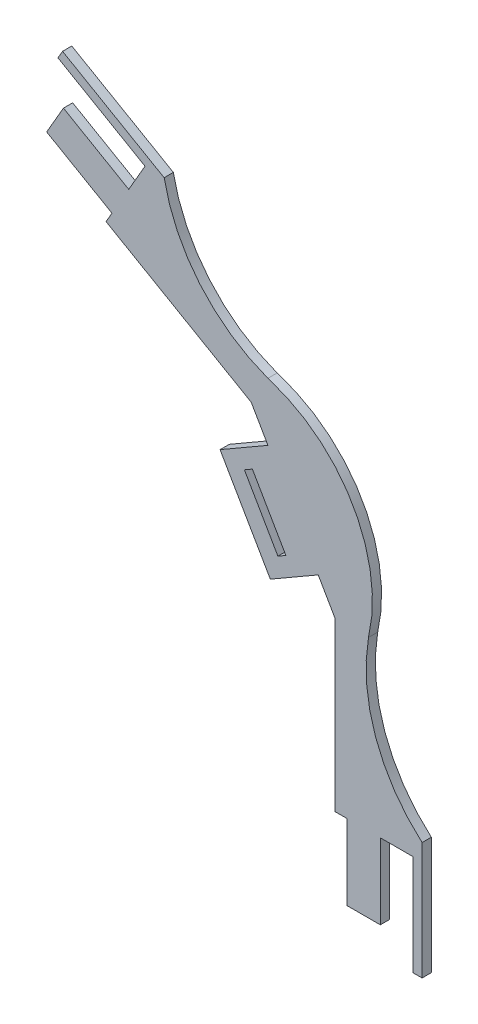
# Autodesk Inventor part: brazos
Saved by Autodesk Inventor 2015 (Build 190159000, 159)
## iProperties
Created: 2017-10-02
Part Number: brazos
Material: Generic
Document SubType Name: Modeling
Designer: macbook
Density: 1 g/cm^3
Appearance: Default
Author: macbook
Autodesk Inventor part; units mm, degrees
ref_plane "YZ Plane" through (0, 0, 0) normal (1, 0, 0) x (0, 1, 0)
ref_plane "XZ Plane" through (0, 0, 0) normal (0, 1, 0) x (-1, 0, 0)
ref_plane "XY Plane" through (0, 0, 0) normal (0, 0, 1) x (1, 0, 0)
sketch "Sketch1" plane through (0, 0, 0) normal (0, 0, 1) x (1, 0, 0)
  arc A0 (20, 100) -> (52, 10) centre (115.8042, 83.3748) ccw
  line L0 (-10, 117.3205) -> (-38.5788, 100.8205)
  line L1 (-38.5788, 100.8205) -> (-68.5788, 152.782)
  line L2 (-68.5788, 152.782) -> (-40, 169.282)
  line L3 (-29.2894, 117.7308) -> (-34.0526, 114.9808)
  line L4 (-34.0526, 114.9808) -> (-54.0526, 149.6218)
  line L5 (-54.0526, 149.6218) -> (-49.2894, 152.3718)
  line L6 (-49.2894, 152.3718) -> (-29.2894, 117.7308)
  line L7 (-136.6025, 236.6025) -> (-50, 186.6025)
  arc A1 (-101.9423, 276.6359) -> (-40, 203.923) centre (-6.4957, 295.2045) ccw
  line L8 (-136.6025, 236.6025) -> (-50, 186.6025)
  arc A2 (20, 100) -> (-40, 203.923) centre (-65.07, 120.1668) ccw
  line L9 (-10, 117.3205) -> (0, 100)
  line L10 (-40, 169.282) -> (-50, 186.6025)
  line L11 (0, 100) -> (0, 0)
  line L12 (52, 10) -> (52, 0)
  line L13 (-110.6025, 281.6359) -> (-101.9423, 276.6359)
  line L14 (46.5, 0) -> (27.071, 0)
  line L15 (7.071, 0) -> (0, 0)
  line L16 (-136.6025, 236.6025) -> (-133.067, 242.7262)
  line L17 (-136.6025, 236.6025) -> (-129.5315, 236.6025) construction
  line L18 (-123.067, 260.0467) -> (-113.3525, 276.8727)
  line L19 (7.071, 0) -> (7.071, -45)
  line L20 (7.071, -45) -> (27.071, -45)
  line L21 (27.071, -45) -> (27.071, 0)
  line L22 (46.5, 0) -> (46.5, -60)
  line L23 (46.5, -60) -> (52, -60)
  line L24 (52, -60) -> (52, 0)
  line L25 (-110.6025, 281.6359) -> (-149.5737, 304.1359)
  line L26 (-152.3237, 299.3727) -> (-113.3525, 276.8727)
  line L27 (-123.067, 260.0467) -> (-162.0382, 282.5467)
  line L28 (-162.0382, 282.5467) -> (-172.0382, 265.2262)
  line L29 (-172.0382, 265.2262) -> (-133.067, 242.7262)
  line L30 (-149.5737, 304.1359) -> (-162.5641, 311.6359)
  line L31 (-162.5641, 311.6359) -> (-165.3141, 306.8727)
  line L32 (-165.3141, 306.8727) -> (-152.3237, 299.3727)
  dimension "d9" = 33
  dimension "d10" = 60
  dimension "d11" = 5.5
  dimension "d12" = 40
  dimension "d13" = 52
  dimension "d14" = 100
  dimension "d28" = 19.429
  dimension "d34" = 60
  dimension "d39" = 19.429
  dimension "d43" = 45
  dimension "d44" = 60
  constraints: 66 end point, 10 perpendicular, 6 point on circle, 4 parallel, 4 vertical, 3 centre point, 3 horizontal, 2 collinear, 1 equal length, 1 point on line
  measures "d9" distance of L1.end L2.end
  measures "d10" distance of L0.end L1.end
  measures "d11" distance of L4.end L5.end
  measures "d12" distance of L3.end L4.end
  measures "d13" distance of L11.end L12.end
  measures "d14" distance of L11.end L9.end
  measures "d28" distance of L14.start L14.end
  measures "d34" angle of L17 L16
  measures "d39" distance of L18.start L18.end
  measures "d43" distance of L15.start L19.end
  measures "d44" distance of L14.start L22.end
extrude "Extrusion2" add sketch "Sketch1" along normal blind 5.5
body "Solid2"
